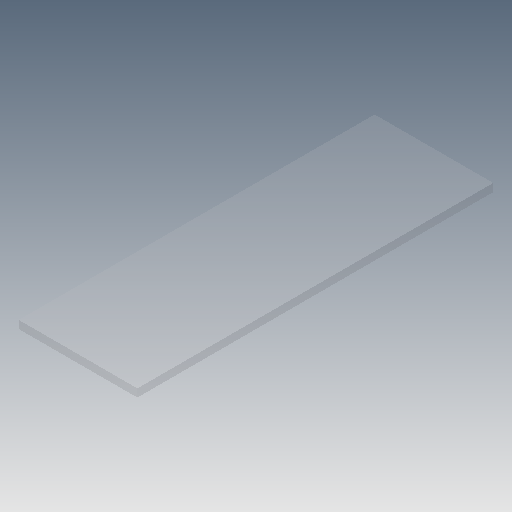
# Autodesk Inventor part: Instrumentation_Frame_SK
Saved by Autodesk Inventor 2019.1 (Build 231200000, 200)
## iProperties
Created: 2009-08-11
Part Number: Instrumentation_Frame_SK
Document SubType Name: Modeling
Designer: Demir Ali
Density: 1 g/cm^3
Mass: 43200 g
Surface Area: 23520 cm^2
Volume: 43200 cm^3
Material: Generic
Description: Instrumentation Frame SK
Stock Number: NA
Appearance: Clear - Light
Title: Manufactured Part
Author: Demir Ali
Revision Number: A
Autodesk Inventor part; units mm, degrees
ref_plane "YZ Plane" through (0, 0, 0) normal (1, 0, 0) x (0, 1, 0)
ref_plane "XZ Plane" through (0, 0, 0) normal (0, 1, 0) x (-1, 0, 0)
ref_plane "XY Plane" through (0, 0, 0) normal (0, 0, 1) x (1, 0, 0)
sketch "Sketch1" plane through (0, 0, 0) normal (0, 0, 1) x (1, 0, 0)
  line L0 (-300, -20) -> (300, -20)
  line L1 (300, -20) -> (300, 20)
  line L2 (300, 20) -> (-300, 20)
  line L3 (-300, 20) -> (-300, -20)
  point P0 (0, 0)
  point P1 (-300, 0)
  point P2 (0, 20)
  dimension "d0" = 40
  dimension "d1" = 600
  constraints: 8 end point, 2 midpoint, 2 parallel, 1 horizontal, 1 horizontal alignment, 1 perpendicular, 1 vertical alignment
  measures "d0" distance of L2.end L0.start
  measures "d1" distance of L1.end L2.end
extrude "Extrusion1" add sketch "Sketch1" along normal blind 1800
sketch "Board_SK" plane through (-300, -20, 0) normal (0, -1, 0) x (1, 0, 0)
  line L0 (600, 1800) -> (0, 1800) projected
  line L1 (0, 0) -> (0, 1800) projected
  line L2 (0, 0) -> (600, 0) projected
  line L3 (600, 0) -> (600, 1800) projected
  line L4 (-75, 1875) -> (675, 1875)
  line L5 (675, 1875) -> (675, 875)
  line L6 (675, 875) -> (-75, 875)
  line L7 (-75, 875) -> (-75, 1875)
  point P0 (300, 0)
  point P1 (300, 1800)
  point P2 (300, 1875)
  dimension "d4" = 75
  dimension "d5" = 75
  dimension "d6" = 1000
  constraints: 8 end point, 2 midpoint, 2 parallel, 1 horizontal, 1 perpendicular, 1 vertical alignment
  measures "d4" distance between parallel lines of L0 L4
  measures "d5" distance between parallel lines of L7 L1
  measures "d6" distance of L6.end L4.start
sketch "Base_SK" plane through (-300, -20, 0) normal (0, -1, 0) x (1, 0, 0)
  line L0 (600, 1800) -> (0, 1800) projected
  line L1 (0, 0) -> (0, 1800) projected
  line L2 (0, 0) -> (600, 0) projected
  line L3 (600, 0) -> (600, 1800) projected
  line L4 (600, 950) -> (0, 950)
  point P0 (300, 0)
  dimension "d7" = 850
  constraints: 2 end point, 2 point on line, 1 perpendicular
  measures "d7" distance between parallel lines of L4 L0
equation "\"d5\" = d4"
equation "\"d7\" = d6 - 2 * d4"
body "Solid1"
